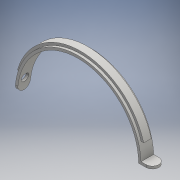
# Autodesk Inventor part: Metal icecream cutter
Saved by Autodesk Inventor 2016 (Build 200138000, 138)
## iProperties
Created: 2016-11-05
Part Number: Metal icecream cutter
Material: Generic
Document SubType Name: Modeling
Designer: Muhammad
Density: 1 g/cm^3
Appearance: Chrome - Polished
Author: Muhammad
Autodesk Inventor part; units mm, degrees
ref_plane "XY Plane" through (0, 0, 0) normal (0, 0, 1) x (1, 0, 0)
sketch "Sketch1" plane through (0, 0, 0) normal (0, 1, 0) x (-1, 0, 0)
  arc A0 (25, 0) -> (-24.98, 1) centre (0, 0) ccw
  arc A1 (24, 0) -> (-24, 0) centre (0, 0) ccw
  line L0 (25, 0) -> (24, 0)
  line L1 (-24, 0) -> (-25, 0)
  line L2 (-24, 0) -> (-29.5, 0)
  line L3 (-29.5, 0) -> (-29.5, 1)
  line L4 (-29.5, 1) -> (-24.98, 1)
  line L5 (-24, 1) -> (-24, 0)
  constraints: 12 end point, 4 point on circle, 2 centre point, 2 coincident, 2 horizontal, 2 parallel, 1 collinear, 1 perpendicular
extrude "Extrusion1" add sketch "Sketch1" along normal blind 5
sketch "Sketch2" plane through (29.5, 0, 0) normal (0, 0, -1) x (-1, 0, 0)
  line L0 (0, 0) -> (5.5, 0) projected
  arc A0 (2.5, 5) -> (2.5, 0) centre (2.5, 2.5) ccw
  line L1 (0, 0) -> (2.5, 0)
  line L2 (4.52, 0) -> (0, 0) projected
  line L3 (0, 0) -> (0, 2.5)
  line L4 (0, 0) -> (0, 5) projected
  line L5 (0, 2.5) -> (0, 5)
  line L6 (0, 5) -> (2.26, 5)
  line L7 (4.52, 5) -> (0, 5) projected
  line L8 (2.5, 5) -> (0, 5)
  line L9 (0, 2.5) -> (0, 5)
  line L10 (0, 2.5) -> (0, 0)
  line L11 (0, 0) -> (2.5, 0)
  arc A1 (0, 2.5) -> (2.5, 0) centre (2.5, 2.5) ccw
  arc A2 (2.5, 5) -> (0, 2.5) centre (2.5, 2.5) ccw
  point P0 (29.5, 0)
  constraints: 16 end point, 6 point on circle, 5 collinear, 5 tangent, 3 centre point, 3 point on line, 2 coincident, 2 midpoint
extrude "Extrusion2" cut sketch "Sketch2" against normal through all
ref_plane "Work Plane1" through (-25, 0, 0) normal (1, 0, 0) x (0, 1, 0)
sketch "Sketch3" plane through (-25, 0, 0) normal (1, 0, 0) x (0, 1, 0)
  line L0 (5, 0) -> (5, 25) construction
  line L1 (0, 0) -> (0, 2) construction
  line L2 (0, 0) -> (0, 25) construction
  line L3 (0, 0) -> (0, 2.5) construction
  arc A0 (0, 2.5) -> (5, 2.5) centre (2.5, 2.5) ccw
  line L4 (0, 0) -> (0, 2.5)
  line L5 (0, 0) -> (5, 0) projected
  line L6 (0, 0) -> (2.5, 0)
  line L7 (2.5, 0) -> (5, 0)
  line L8 (5, 0) -> (5, 2.5)
  arc A1 (0, 2.5) -> (2.5, 0) centre (2.5, 2.5) ccw
  arc A2 (2.5, 0) -> (5, 2.5) centre (2.5, 2.5) ccw
  point P0 (0, 1)
  point P1 (5, 1)
  constraints: 12 end point, 6 point on circle, 3 centre point, 2 coincident, 2 collinear, 2 point on line, 1 midpoint, 1 tangent
extrude "Extrusion3" cut sketch "Sketch3" along normal blind 3
sketch "Sketch4" plane through (-25, 0, 0) normal (1, 0, 0) x (0, 1, 0)
  line L0 (0, 0) -> (0, 4.5) construction
  line L1 (0, 24) -> (0, 0) construction
  line L2 (0, 4.5) -> (5, 4.5) construction
  line L3 (5, 24) -> (5, 0) construction
  circle A0 centre (2.5, 4.5) radius 1.5
  point P0 (0, 2.5)
  point P1 (5, 2.5)
  dimension "d15" = 4.5
  dimension "d16" = 3
  constraints: 4 end point, 2 point on line, 1 centre point, 1 midpoint, 1 perpendicular
  measures "d15" distance of L0.start L0.end
  measures "d16" diameter of A0
extrude "Extrusion4" cut sketch "Sketch4" along normal blind 4
ref_plane "Work Plane2" through (0, 2.5, 0) normal (0, 1, 0) x (-1, 0, 0)
sketch "Sketch6" plane through (0, 2.5, 0) normal (0, 1, 0) x (-1, 0, 0)
  arc A0 (25.04, 7) -> (-25.04, 7) centre (0, 0) ccw
  line L0 (23.9792, 7) -> (25.04, 7)
  line L1 (-23.9792, 7) -> (-25.04, 7)
  arc A1 (23.9792, 7) -> (-23.9792, 7) centre (0, 0) ccw
  point P0 (0, 7)
  dimension "d22" = 52
  dimension "d23" = 7
  constraints: 4 end point, 4 point on circle, 2 centre point, 2 horizontal, 1 coincident
  measures "d22" diameter of A0
  measures "d23" distance of A0.centre point (0, 7)
extrude "Extrusion5" add sketch "Sketch6" along normal mid plane 3
body "Solid1"
